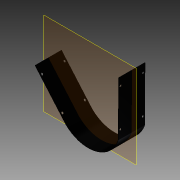
# Autodesk Inventor part: Sheild
Saved by Autodesk Inventor 2013 (Build 170138000, 138)
## iProperties
Created: 2013-06-27
Part Number: Sheild
Material: Generic
Document SubType Name: Modeling
Designer: mvarma
Density: 1 g/cm^3
Author: mvarma
Autodesk Inventor part; units mm, degrees
ref_plane "YZ Plane" through (0, 0, 0) normal (1, 0, 0) x (0, 1, 0)
ref_plane "XZ Plane" through (0, 0, 0) normal (0, 1, 0) x (-1, 0, 0)
ref_plane "XY Plane" through (0, 0, 0) normal (0, 0, 1) x (1, 0, 0)
sketch "Sketch1" plane through (0, 0, 0) normal (0, 0, 1) x (1, 0, 0)
  arc A0 (67.8806, 113.5366) -> (74.024, 136.5789) centre (56.3452, 128.9522) ccw construction
  line L0 (63.0849, 61.9574) -> (112.0151, 5.0878)
  arc A1 (67.8806, 113.5366) -> (63.0849, 61.9574) centre (88.8014, 85.5789) ccw construction
  arc A2 (139.2877, 161.4802) -> (160.6194, 146.2689) centre (160.3908, 168.5113) ccw construction
  arc A3 (170.156, 145.0434) -> (160.6194, 146.2689) centre (160.9785, 111.3458) ccw construction
  line L1 (195.9029, 111.1496) -> (195.4212, 25.3733)
  ellipse E0 centre (106.1636, 150.4439) end of major axis (106.1759, 186.8392) minor radius 34.7604 (139.2877, 161.4802) -> (74.024, 136.5789) ccw construction
  arc A4 (112.0151, 5.0878) -> (112.3757, 4.7043) centre (116.5302, 8.9726) ccw
  arc A5 (112.3757, 4.7043) -> (195.1395, 23.7862) centre (147.6111, 40.9044) ccw
  arc A6 (195.1395, 23.7862) -> (195.4212, 25.3733) centre (190.6588, 25.4) ccw
  arc A7 (195.9029, 111.1496) -> (170.156, 145.0434) centre (160.9785, 111.3458) ccw construction
  line L2 (111.4134, 4.5701) -> (62.4916, 61.4299)
  arc A8 (67.4051, 114.1722) -> (62.4916, 61.4299) centre (88.8014, 85.5789) ccw construction
  arc A9 (67.4051, 114.1722) -> (73.2902, 136.2761) centre (56.3452, 128.9522) ccw construction
  arc A10 (140.0441, 161.7212) -> (160.6113, 147.0626) centre (160.3908, 168.5113) ccw construction
  arc A11 (170.3646, 145.8092) -> (160.6113, 147.0626) centre (160.9785, 111.3458) ccw construction
  arc A12 (196.6967, 111.1452) -> (170.3646, 145.8092) centre (160.9785, 111.3458) ccw construction
  line L3 (196.6967, 111.1452) -> (196.2149, 25.3688)
  arc A13 (195.8863, 23.5172) -> (196.2149, 25.3688) centre (190.6588, 25.4) ccw
  arc A14 (111.8221, 4.1355) -> (195.8863, 23.5172) centre (147.6111, 40.9044) ccw
  arc A15 (111.4134, 4.5701) -> (111.8221, 4.1355) centre (116.5302, 8.9726) ccw
  line L4 (63.0849, 61.9574) -> (62.4916, 61.4299)
  line L5 (195.9029, 111.1496) -> (196.6967, 111.1452)
  spline S0 degree 5 poles (73.2902, 136.2761) (72.7058, 137.7596) (72.1989, 139.2737) (71.7711, 140.8127) (70.2947, 147.4301) (70.2772, 154.2953) (71.1378, 159.497) (74.5342, 169.3198) (80.981, 177.4616) (84.8447, 180.9023) (93.5768, 186.2035) (103.6086, 188.0948) (108.7095, 188.0956) (118.7418, 186.2077) (127.4753, 180.9092) (131.3399, 177.4697) (135.5266, 172.185) (138.4279, 166.1913) (139.0439, 164.7287) (139.583, 163.2368) (140.0441, 161.7212) knots 0 0 0 0 0 0 0.067943 0.067943 0.067943 0.288528 0.288528 0.288528 0.504379 0.504379 0.504379 0.716654 0.716654 0.716654 0.932497 0.932497 0.932497 1 1 1 1 1 1 construction
  point P0 (0, 0)
  point P1 (93.6139, 184.384)
  point P2 (71.7596, 145.2447)
  point P3 (61.2825, 107.0736)
  point P4 (135.0639, 170.6681)
  point P5 (195.5971, 56.6944)
  point P6 (88.1705, 44.9716)
  dimension "d0" = 0.7937
  constraints: 33 point on circle, 16 centre point, 12 end point, 2 coincident, 2 concentric, 2 tangent, 1 perpendicular, 1 point on line, 56 other
  measures "d0" distance between parallel lines of L2 L0
extrude "Extrusion1" add sketch "Sketch1" along normal blind 42.164
sketch "Sketch2" plane through (195.4212, 25.3733, 0) normal (-0.9999842, 0.0056163, 0) x (0, 0, 1)
  line L0 (0, 0) -> (42.164, 0) projected
  line L1 (42.164, 85.7777) -> (42.164, 0) projected
  line L2 (0, 85.7777) -> (42.164, 85.7777) projected
  line L3 (38.989, 85.7777) -> (38.989, 0) construction
  point P0 (0, -26.4704)
  point P1 (38.989, 73.0777)
  point P2 (38.989, 12.7)
  dimension "d4" = 3.175
  dimension "d5" = 12.7
  dimension "d6" = 12.7
  constraints: 4 point on line, 2 end point, 1 perpendicular
  measures "d4" distance between parallel lines of L1 L3
  measures "d5" distance from line of L2 point (38.989, 73.078)
  measures "d6" distance from line of L0 point (38.989, 12.7)
hole "Hole1" at (195.8316, 98.4498, 38.989) at (195.4925, 38.0731, 38.989) direction (0.9999842, -0.0056163, 0) diameter 3.2766 end through all clearance for "Flat Head Machine Screw (82)" size "#4" standard "Ansi Unified Screw Threads"
sketch "Sketch3" plane through (63.0849, 61.9574, 42.164) normal (0.758038, 0.6522104, 0) x (0, 0, -1)
  line L0 (42.164, 0) -> (0, 0) projected
  line L1 (0, -75.022) -> (0, 0) projected
  line L2 (42.164, -75.022) -> (0, -75.022) projected
  line L3 (3.175, 0) -> (3.175, -75.022) construction
  point P0 (42.164, -5.8214)
  point P1 (3.175, -62.322)
  point P2 (3.175, -12.7)
  dimension "d14" = 3.175
  dimension "d15" = 12.7
  dimension "d16" = 12.7
  constraints: 4 point on line, 2 end point, 1 perpendicular
  measures "d14" distance between parallel lines of L1 L3
  measures "d15" distance from line of L0 point (3.175, -12.7)
  measures "d16" distance from line of L2 point (3.175, -62.322)
hole "Hole2" at (103.732, 14.7149, 38.989) at (71.368, 52.3303, 38.989) direction (-0.758038, -0.6522104, 0) diameter 3.2766 depth 25.4 tip angle 118 clearance for "Flat Head Machine Screw (82)" size "#4" standard "Ansi Unified Screw Threads"
ref_plane "Mid Plane" through (0, 0, 21.082) normal (0, 0, 1) x (1, 0, 0)
mirror "Mirror1" about plane through (0, 0, 21.082) normal (0, 0, 1) of "Hole1", "Hole2"
body "Solid1"
